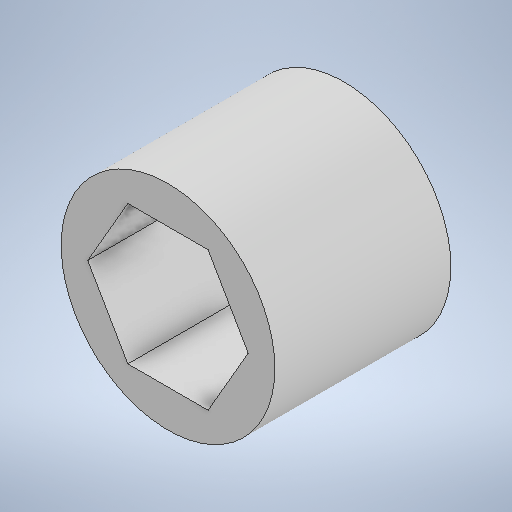
# Autodesk Inventor part: 0.633 Spacer 0.5 Hex
Saved by Autodesk Inventor 2025.1 (Build 291241020, 241B)
## iProperties
Created: 2024-10-06
Part Number: 0.633 Spacer 0.5 Hex
Material: Generic
Document SubType Name: Modeling
Designer: xmand
Density: 1 g/cm^3
Appearance: Default
Author: xmand
Autodesk Inventor part; units mm, degrees
ref_plane "YZ Plane" through (0, 0, 0) normal (1, 0, 0) x (0, 1, 0)
ref_plane "XZ Plane" through (0, 0, 0) normal (0, 1, 0) x (-1, 0, 0)
ref_plane "XY Plane" through (0, 0, 0) normal (0, 0, 1) x (1, 0, 0)
sketch "Sketch1" plane through (0, 0, 0) normal (0, 0, 1) x (1, 0, 0)
  line L0 (7.3293, 0) -> (3.6646, -6.3473)
  line L1 (3.6646, -6.3473) -> (-3.6646, -6.3473)
  line L2 (-3.6646, -6.3473) -> (-7.3293, 0)
  line L3 (-7.3293, 0) -> (-3.6646, 6.3473)
  line L4 (-3.6646, 6.3473) -> (3.6646, 6.3473)
  line L5 (3.6646, 6.3473) -> (7.3293, 0)
  circle A0 centre (0, 0) radius 9.7536
  dimension "d0" = 19.5072
  dimension "d1" = 12.6947
  constraints: 12 end point, 2 coincident, 1 centre point, 1 horizontal, 13 other
  measures "d0" diameter of A0
  measures "d1" distance between parallel lines of L1 L4
extrude "Extrusion1" add sketch "Sketch1" along normal mid plane 16.0782
body "Solid1"
